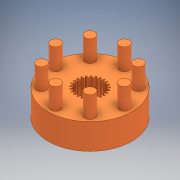
# Autodesk Inventor part: moto_gear
Saved by Autodesk Inventor 2018 (Build 220112000, 112)
## iProperties
Created: 2019-01-07
Part Number: moto_gear
Material: 一般
Document SubType Name: Modeling
Designer: lowyu
Density: 1 g/cm^3
Appearance: 既定
Author: lowyu
Autodesk Inventor part; units mm, degrees
ref_plane "YZ Plane" through (0, 0, 0) normal (1, 0, 0) x (0, 1, 0)
ref_plane "XZ Plane" through (0, 0, 0) normal (0, 1, 0) x (-1, 0, 0)
ref_plane "XY Plane" through (0, 0, 0) normal (0, 0, 1) x (1, 0, 0)
sketch "スケッチ1" plane through (0, 0, 0) normal (0, 0, 1) x (1, 0, 0)
  circle A0 centre (0, 0) radius 9.75
  constraints: 1 centre point
extrude "押し出し1" add sketch "スケッチ1" along normal blind 6
sketch "スケッチ4" plane through (0, 0, 6) normal (0, 0, 1) x (1, 0, 0)
  circle A0 centre (-5.6569, 5.6569) radius 1.15
  circle A1 centre (-8, 0) radius 1.15
  circle A2 centre (-5.6569, -5.6569) radius 1.15
  circle A3 centre (0, -8) radius 1.15
  circle A4 centre (5.6569, -5.6569) radius 1.15
  circle A5 centre (0, 8) radius 1.15
  circle A6 centre (5.6569, 5.6569) radius 1.15
  circle A7 centre (8, 0) radius 1.15
  point P0 (0, 0)
  point P1 (0, 0)
  constraints: 8 centre point
extrude "押し出し4" add sketch "スケッチ4" along normal blind 5
sketch "スケッチ6" plane through (0, 0, 0) normal (0, 0, -1) x (-1, 0, 0)
  arc A0 (-0.9924, 3.2258) -> (-0.9924, 2.6305) centre (0.2216, 2.9282) ccw
  arc A1 (-0.8525, 3.2656) -> (-0.9924, 3.2258) centre (0, 0) ccw
  arc A2 (-0.5394, 2.7593) -> (-0.8525, 3.2656) centre (-1.7285, 2.3739) ccw
  arc A3 (-0.307, 2.7947) -> (-0.5394, 2.7593) centre (0, 0) ccw
  arc A4 (-0.159, 3.3713) -> (-0.307, 2.7947) centre (0.9429, 2.781) ccw
  arc A5 (-0.0136, 3.375) -> (-0.159, 3.3713) centre (0, 0) ccw
  arc A6 (0.1637, 2.8067) -> (-0.0136, 3.375) centre (-1.0839, 2.7292) ccw
  arc A7 (0.3976, 2.7832) -> (0.1637, 2.8067) centre (0, 0) ccw
  arc A8 (0.6844, 3.3049) -> (0.3976, 2.7832) centre (1.6049, 2.4592) ccw
  arc A9 (0.8261, 3.2723) -> (0.6844, 3.3049) centre (0, 0) ccw
  arc A10 (0.8566, 2.6778) -> (0.8261, 3.2723) centre (-0.3711, 2.913) ccw
  arc A11 (1.0773, 2.5969) -> (0.8566, 2.6778) centre (0, 0) ccw
  arc A12 (1.4848, 3.0308) -> (1.0773, 2.5969) centre (2.166, 1.9828) ccw
  arc A13 (1.614, 2.9641) -> (1.4848, 3.0308) centre (0, 0) ccw
  arc A14 (1.4956, 2.3807) -> (1.614, 2.9641) centre (0.365, 2.9138) ccw
  arc A15 (1.6893, 2.2474) -> (1.4956, 2.3807) centre (0, 0) ccw
  arc A16 (2.1919, 2.5664) -> (1.6893, 2.2474) centre (2.5911, 1.3818) ccw
  arc A17 (2.3004, 2.4696) -> (2.1919, 2.5664) centre (0, 0) ccw
  arc A18 (2.0407, 1.9339) -> (2.3004, 2.4696) centre (1.0782, 2.7315) ccw
  arc A19 (2.1951, 1.7567) -> (2.0407, 1.9339) centre (0, 0) ccw
  arc A20 (2.7612, 1.9407) -> (2.1951, 1.7567) centre (2.8533, 0.6941) ccw
  arc A21 (2.8423, 1.8199) -> (2.7612, 1.9407) centre (0, 0) ccw
  arc A22 (2.4575, 1.3657) -> (2.8423, 1.8199) centre (1.7236, 2.3775) ccw
  arc A23 (2.563, 1.1556) -> (2.4575, 1.3657) centre (0, 0) ccw
  arc A24 (3.1571, 1.193) -> (2.563, 1.1556) centre (2.9363, -0.0374) ccw
  arc A25 (3.2056, 1.0559) -> (3.1571, 1.193) centre (0, 0) ccw
  arc A26 (2.72, 0.7116) -> (3.2056, 1.0559) centre (2.2607, 1.8742) ccw
  arc A27 (2.7699, 0.4819) -> (2.72, 0.7116) centre (0, 0) ccw
  arc A28 (3.3546, 0.3704) -> (2.7699, 0.4819) centre (2.8348, -0.7664) ccw
  arc A29 (3.3675, 0.2255) -> (3.3546, 0.3704) centre (0, 0) ccw
  arc A30 (2.8115, 0.0128) -> (3.3675, 0.2255) centre (2.6558, 1.2531) ccw
  arc A31 (2.8027, -0.2221) -> (2.8115, 0.0128) centre (0, 0) ccw
  arc A32 (3.3413, -0.4755) -> (2.8027, -0.2221) centre (2.5551, -1.4473) ccw
  arc A33 (3.3177, -0.619) -> (3.3413, -0.4755) centre (0, 0) ccw
  arc A34 (2.7263, -0.6868) -> (3.3177, -0.619) centre (2.8839, 0.5533) ccw
  arc A35 (2.6594, -0.9121) -> (2.7263, -0.6868) centre (0, 0) ccw
  arc A36 (3.1181, -1.2915) -> (2.6594, -0.9121) centre (2.1149, -2.0373) ccw
  arc A37 (3.0596, -1.4247) -> (3.1181, -1.2915) centre (0, 0) ccw
  arc A38 (2.4699, -1.3432) -> (3.0596, -1.4247) centre (2.9309, -0.1813) ccw
  arc A39 (2.3491, -1.5448) -> (2.4699, -1.3432) centre (0, 0) ccw
  arc A40 (2.6989, -2.0264) -> (2.3491, -1.5448) centre (1.5418, -2.4992) ccw
  arc A41 (2.6091, -2.1408) -> (2.6989, -2.0264) centre (0, 0) ccw
  arc A42 (2.0583, -1.9152) -> (2.6091, -2.1408) centre (2.7938, -0.9045) ccw
  arc A43 (1.8911, -2.0805) -> (2.0583, -1.9152) centre (0, 0) ccw
  arc A44 (2.1102, -2.6339) -> (1.8911, -2.0805) centre (0.8718, -2.8041) ccw
  arc A45 (1.9948, -2.7224) -> (2.1102, -2.6339) centre (0, 0) ccw
  arc A46 (1.5173, -2.3669) -> (1.9948, -2.7224) centre (2.481, -1.5709) ccw
  arc A47 (1.3143, -2.4854) -> (1.5173, -2.3669) centre (0, 0) ccw
  arc A48 (1.3889, -3.076) -> (1.3143, -2.4854) centre (0.1471, -2.9329) ccw
  arc A49 (1.2551, -3.133) -> (1.3889, -3.076) centre (0, 0) ccw
  arc A50 (0.881, -2.6699) -> (1.2551, -3.133) centre (2.0124, -2.1385) ccw
  arc A51 (0.6549, -2.7342) -> (0.881, -2.6699) centre (0, 0) ccw
  arc A52 (0.5803, -3.3247) -> (0.6549, -2.7342) centre (-0.5869, -2.8773) ccw
  arc A53 (0.4365, -3.3467) -> (0.5803, -3.3247) centre (0, 0) ccw
  arc A54 (0.1893, -2.8051) -> (0.4365, -3.3467) centre (1.4174, -2.5718) ccw
  arc A55 (-0.0457, -2.8111) -> (0.1893, -2.8051) centre (0, 0) ccw
  arc A56 (-0.2648, -3.3646) -> (-0.0457, -2.8111) centre (-1.284, -2.6409) ccw
  arc A57 (-0.4095, -3.3501) -> (-0.2648, -3.3646) centre (0, 0) ccw
  arc A58 (-0.5142, -2.7641) -> (-0.4095, -3.3501) centre (0.7333, -2.8435) ccw
  arc A59 (-0.7433, -2.7115) -> (-0.5142, -2.7641) centre (0, 0) ccw
  arc A60 (-1.0932, -3.193) -> (-0.7433, -2.7115) centre (-1.9004, -2.2387) ccw
  arc A61 (-1.2298, -3.143) -> (-1.0932, -3.193) centre (0, 0) ccw
  arc A62 (-1.1855, -2.5494) -> (-1.2298, -3.143) centre (0.0031, -2.9365) ccw
  arc A63 (-1.3943, -2.4414) -> (-1.1855, -2.5494) centre (0, 0) ccw
  arc A64 (-1.8529, -2.8209) -> (-1.3943, -2.4414) centre (-2.3975, -1.6957) ccw
  arc A65 (-1.9728, -2.7384) -> (-1.8529, -2.8209) centre (0, 0) ccw
  arc A66 (-1.7822, -2.1745) -> (-1.9728, -2.7384) centre (-0.7273, -2.845) ccw
  arc A67 (-1.9576, -2.018) -> (-1.7822, -2.1745) centre (0, 0) ccw
  arc A68 (-2.4962, -2.2714) -> (-1.9576, -2.018) centre (-2.7439, -1.0462) ccw
  arc A69 (-2.5918, -2.1618) -> (-2.4962, -2.2714) centre (0, 0) ccw
  arc A70 (-2.267, -1.6629) -> (-2.5918, -2.1618) centre (-1.412, -2.5748) ccw
  arc A71 (-2.398, -1.4677) -> (-2.267, -1.6629) centre (0, 0) ccw
  arc A72 (-2.9827, -1.5793) -> (-2.398, -1.4677) centre (-2.9178, -0.331) ccw
  arc A73 (-3.048, -1.4493) -> (-2.9827, -1.5793) centre (0, 0) ccw
  arc A74 (-2.6093, -1.0469) -> (-3.048, -1.4493) centre (-2.008, -2.1427) ccw
  arc A75 (-2.6877, -0.8253) -> (-2.6093, -1.0469) centre (0, 0) ccw
  arc A76 (-3.2817, -0.7879) -> (-2.6877, -0.8253) centre (-2.9085, 0.4051) ccw
  arc A77 (-3.3126, -0.6458) -> (-3.2817, -0.7879) centre (0, 0) ccw
  arc A78 (-2.7877, -0.3651) -> (-3.3126, -0.6458) centre (-2.4778, -1.5761) ccw
  arc A79 (-2.8084, -0.131) -> (-2.7877, -0.3651) centre (0, 0) ccw
  arc A80 (-3.3746, 0.053) -> (-2.8084, -0.131) centre (-2.7164, 1.1157) ccw
  arc A81 (-3.3692, 0.1983) -> (-3.3746, 0.053) centre (0, 0) ccw
  arc A82 (-2.7909, 0.3396) -> (-3.3692, 0.1983) centre (-2.7919, -0.9104) ccw
  arc A83 (-2.7528, 0.5716) -> (-2.7909, 0.3396) centre (0, 0) ccw
  arc A84 (-3.2554, 0.8906) -> (-2.7528, 0.5716) centre (-2.3536, 1.7561) ccw
  arc A85 (-3.214, 1.03) -> (-3.2554, 0.8906) centre (0, 0) ccw
  arc A86 (-2.6188, 1.023) -> (-3.214, 1.03) centre (-2.9306, -0.1875) ccw
  arc A87 (-2.5241, 1.2382) -> (-2.6188, 1.023) centre (0, 0) ccw
  arc A88 (-2.9316, 1.6722) -> (-2.5241, 1.2382) centre (-1.8429, 2.2863) ccw
  arc A89 (-2.8569, 1.7969) -> (-2.9316, 1.6722) centre (0, 0) ccw
  arc A90 (-2.2821, 1.6422) -> (-2.8569, 1.7969) centre (-2.8851, 0.5472) ccw
  arc A91 (-2.1369, 1.8271) -> (-2.2821, 1.6422) centre (0, 0) ccw
  arc A92 (-2.4237, 2.3487) -> (-2.1369, 1.8271) centre (-1.2164, 2.6727) ccw
  arc A93 (-2.3202, 2.4509) -> (-2.4237, 2.3487) centre (0, 0) ccw
  arc A94 (-1.802, 2.1581) -> (-2.3202, 2.4509) centre (-2.6584, 1.2475) ccw
  arc A95 (-1.6154, 2.3011) -> (-1.802, 2.1581) centre (0, 0) ccw
  arc A96 (-1.7634, 2.8777) -> (-1.6154, 2.3011) centre (-0.5135, 2.8913) ccw
  arc A97 (-1.6378, 2.951) -> (-1.7634, 2.8777) centre (0, 0) ccw
  arc A98 (-1.2087, 2.5384) -> (-1.6378, 2.951) centre (-2.2646, 1.8695) ccw
  arc A99 (-0.9924, 2.6305) -> (-1.2087, 2.5384) centre (0, 0) ccw
  constraints: 200 point on circle, 100 centre point, 2 coincident
extrude "押し出し5" cut sketch "スケッチ6" against normal blind 6
